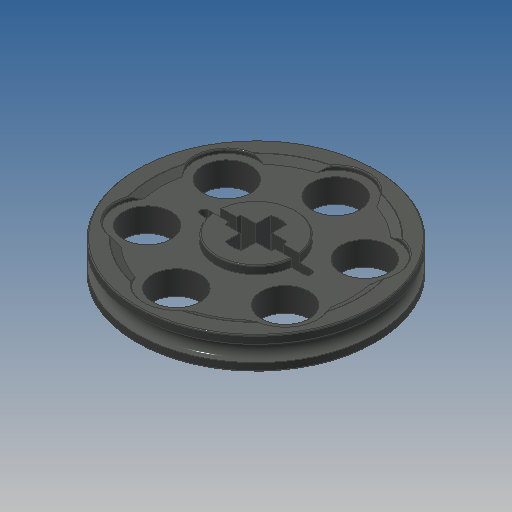
# Autodesk Inventor part: 4185-DkBluishGray
Saved by Autodesk Inventor 2022.2 (Build 262287000, 287)
## iProperties
Created: 2014-10-03
Part Number: 4185-DkBluishGray
Material: ABS Plastic
Document SubType Name: Modeling
Designer: D. Kohfeld
Density: 1.06 g/cm^3
Appearance: DkBluishGray
Mass: 0.903585 g
Surface Area: 13.4553 cm^2
Volume: 0.852439 cm^3
Author: D. Kohfeld
Autodesk Inventor part; units mm, degrees
ref_plane "YZ Plane" through (0, 0, 0) normal (1, 0, 0) x (0, 1, 0)
ref_plane "XZ Plane" through (0, 0, 0) normal (0, 1, 0) x (-1, 0, 0)
ref_plane "XY Plane" through (0, 0, 0) normal (0, 0, 1) x (1, 0, 0)
sketch "Sketch2" plane through (0, 0, 0) normal (0, 0, 1) x (1, 0, 0)
  line L0 (0, -2) -> (0, 2)
  line L1 (0, 2) -> (4, 2)
  line L2 (4, 2) -> (4, 1.2)
  line L3 (4, 1.2) -> (9.6, 1.2)
  line L4 (9.6, 1.2) -> (10.4, 1.6)
  line L5 (10.4, 1.6) -> (12, 1.6)
  line L6 (0, -2) -> (4, -2)
  line L7 (4, -2) -> (4, -1.2)
  line L8 (4, -1.2) -> (9.6, -1.2)
  line L9 (9.6, -1.2) -> (10.4, -1.6)
  line L10 (10.4, -1.6) -> (12, -1.6)
  line L11 (12, -1.6) -> (12, -0.8)
  arc A0 (12, 0.8) -> (12, -0.8) centre (12, 0) ccw
  line L12 (12, 0.8) -> (12, 1.6)
  point P0 (0, 0)
  point P1 (0, 0)
  dimension "d0" = 4
  dimension "d1" = 24
  dimension "d2" = 8
  dimension "d3" = 2.4
  dimension "d4" = 19.2
  dimension "d5" = 20.8
  dimension "d6" = 1.6
  dimension "d7" = 3.2
  constraints: 26 end point, 8 parallel, 4 vertical alignment, 2 collinear, 2 perpendicular, 2 point on circle, 1 centre point, 1 coincident, 1 horizontal alignment, 1 midpoint, 1 point on line, 1 vertical
  measures "d0" distance of L0.start L0.end
  measures "d1" diameter of L5.end L0
  measures "d2" diameter of L1.end L0
  measures "d3" distance between parallel lines of L8 L3
  measures "d4" diameter of L3.end L0
  measures "d5" diameter of L4.end L0
  measures "d6" distance of L11.end L12.start
  measures "d7" distance between parallel lines of L10 L5
revolve "Revolution1" add sketch "Sketch2" angle 360 about axis through (0, -2, 0) along (0, 1, 0)
sketch "Sketch3" plane through (0, 2, 0) normal (0, 1, 0) x (1, 0, 0)
  circle A0 centre (0, 0) radius 4 projected
  circle A1 centre (0, 8) radius 2.4
  circle A2 centre (0, 8) radius 3.2
  circle A3 centre (0, 0) radius 2.4 construction
  line L0 (-0.8, 2.2627) -> (-0.8, 0.8)
  line L1 (-0.8, 0.8) -> (-2.2627, 0.8)
  line L2 (-2.2627, -0.8) -> (-0.8, -0.8)
  line L3 (-0.8, -0.8) -> (-0.8, -2.2627)
  line L4 (0.8, -2.2627) -> (0.8, -0.8)
  line L5 (0.8, -0.8) -> (2.2627, -0.8)
  line L6 (2.2627, 0.8) -> (0.8, 0.8)
  line L7 (0.8, 0.8) -> (0.8, 2.2627)
  arc A4 (0.8, 2.2627) -> (-0.8, 2.2627) centre (0, 0) ccw
  arc A5 (-0.8, -2.2627) -> (0.8, -2.2627) centre (0, 0) ccw
  line L8 (2.3664, -0.4) -> (5.2, -0.4)
  arc A6 (5.2, -0.4) -> (5.2, 0.4) centre (5.2, 0) ccw
  line L9 (5.2, 0.4) -> (2.3664, 0.4)
  line L10 (-2.3664, 0.4) -> (-5.2, 0.4)
  arc A7 (-5.2, 0.4) -> (-5.2, -0.4) centre (-5.2, 0) ccw
  line L11 (-5.2, -0.4) -> (-2.3664, -0.4)
  arc A8 (-2.2627, 0.8) -> (-2.3664, 0.4) centre (0, 0) ccw
  arc A9 (-2.3664, -0.4) -> (-2.2627, -0.8) centre (0, 0) ccw
  arc A10 (2.2627, -0.8) -> (2.3664, -0.4) centre (0, 0) ccw
  arc A11 (2.3664, 0.4) -> (2.2627, 0.8) centre (0, 0) ccw
  dimension "d12" = 4.8
  dimension "d9" = 4.8
  dimension "d10" = 6.4
  dimension "d11" = 8
  dimension "d13" = 1.6
  dimension "d14" = 11.2
  dimension "d15" = 0.8
  constraints: 24 end point, 16 point on circle, 14 equal length, 10 centre point, 5 perpendicular, 4 tangent, 2 coincident, 2 horizontal alignment, 1 equal radius, 1 vertical, 1 vertical alignment, 20 other
  measures "d9" diameter of A1
  measures "d10" diameter of A2
  measures "d11" distance of A1.centre A0.centre
  measures "d13" distance between parallel lines of L7 L0
  measures "d15" distance between parallel lines of L9 L8
extrude "Extrusion1" cut sketch "Sketch3" against normal through all contours A0 L8 A10 L5 L4 A5 L3 L2 A9 L11 L10 A8 L1 L0 A4 L7 L6 A11 L9 | A0 L9 A6 L8 | A0 L11 A7 L10
extrude "Extrusion2" cut sketch "Sketch3" against normal through all contours A1
extrude "Extrusion3" cut sketch "Sketch3" against normal up to surface (0.8 mm away) contours A2
mirror "Mirror1" about plane through (0, 0, 0) normal (0, 1, 0) of "Extrusion3"
pattern_circular "Circular Pattern1" count 6 over 360 about axis through (0, -1.6, 0) along (0, -1, 0) of "Extrusion2", "Extrusion3", "Mirror1"
fillet "Fillet1" radius 0.1 30 edges at (0, 2, 4) (0, 2, -4) (-10.4, 1.6, 0) (-9.6995, 1.6, -5.6) (-12, 1.6, 0) (-12, -1.6, 0) (-5.2, 1.6, 9.0067) (-9.6995, 1.6, 5.6) (-5.2, 1.6, -9.0067) (0, 1.6, -11.2) (5.2, 1.6, -9.0067) (9.6995, 1.6, -5.6) (10.4, 1.6, 0) (9.6995, 1.6, 5.6) (5.2, 1.6, 9.0067) (0, 1.6, 11.2) (-10.4, -1.6, 0) (-9.6995, -1.6, -5.6) (-5.2, -1.6, -9.0067) (0, -1.6, -11.2) (5.2, -1.6, -9.0067) (9.6995, -1.6, -5.6) (10.4, -1.6, 0) (9.6995, -1.6, 5.6) (5.2, -1.6, 9.0067) (0, -1.6, 11.2) (-5.2, -1.6, 9.0067) (-9.6995, -1.6, 5.6) (0, -2, 4) (0, -2, -4)
equation "\"d0\" = 0.5 * lu"
equation "\"d1\" = 3 * lu"
equation "\"d2\" = lu"
equation "\"d6\" = wall"
equation "\"d12\" = kd"
equation "\"d9\" = tpd"
equation "\"d11\" = lu"
equation "\"d13\" = axlet"
equation "\"lu\" = 8"
equation "\"wall\" = 1.6"
equation "\"kd\" = 4.8"
equation "\"tpd\" = 4.8"
equation "\"axlet\" = 1.6"
body "Solid1"
